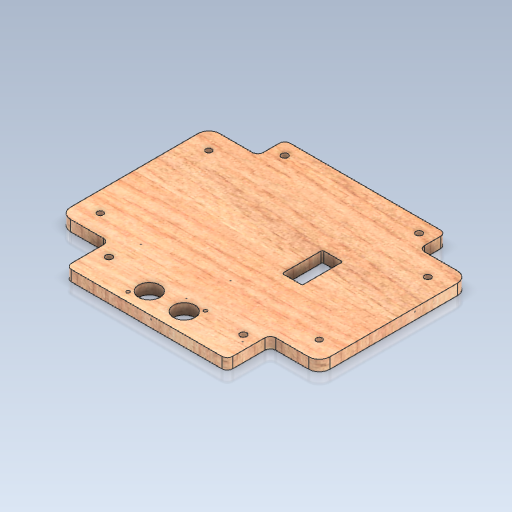
# Autodesk Inventor part: lcd mount back
Saved by Autodesk Inventor 2020.2 (Build 242310000, 310)
## iProperties
Created: 2019-10-18
Part Number: lcd mount back
Material: Wood (Birch)
Document SubType Name: Modeling
Designer: Stefan de Kraker
Density: 0.55 g/cm^3
Appearance: Birch - Natural Polished
Author: Stefan de Kraker
Autodesk Inventor part; units mm, degrees
ref_plane "YZ Plane" through (0, 0, 0) normal (1, 0, 0) x (0, 1, 0)
ref_plane "XZ Plane" through (0, 0, 0) normal (0, 1, 0) x (-1, 0, 0)
ref_plane "XY Plane" through (0, 0, 0) normal (0, 0, 1) x (1, 0, 0)
sketch "Sketch1" plane through (0, 0, 0) normal (0, 1, 0) x (-1, 0, 0)
  arc A0 (0, 0) -> (-7.88, -7.88) centre (0, -7.88) ccw
  line L0 (177.2, 0) -> (0, 0)
  arc A1 (185.08, -7.88) -> (177.2, 0) centre (177.2, -7.88) ccw
  arc A2 (177.2, -110.76) -> (185.08, -102.88) centre (177.2, -102.88) ccw
  line L1 (185.08, -102.88) -> (185.08, -7.88)
  line L2 (0, -110.76) -> (177.2, -110.76)
  line L3 (-7.88, -7.88) -> (-7.88, -102.88)
  arc A3 (-7.88, -102.88) -> (0, -110.76) centre (0, -102.88) ccw
  line L4 (63.5998, -43.83) -> (48.5998, -43.83)
  line L5 (48.5998, -43.83) -> (48.5998, -73.83)
  line L6 (48.5998, -73.83) -> (63.5998, -73.83)
  line L7 (63.5998, -73.83) -> (63.5998, -43.83)
  line L8 (138.6, 10) -> (38.6, 10)
  line L9 (38.6, 10) -> (38.6, -120.76)
  line L10 (38.6, -120.76) -> (138.6, -120.76)
  line L11 (138.6, -120.76) -> (138.6, 10)
  line L12 (148.6, 20) -> (28.6, 20)
  line L13 (28.6, 20) -> (28.6, -130.76)
  line L14 (28.6, -130.76) -> (148.6, -130.76)
  line L15 (148.6, -130.76) -> (148.6, 20)
  line L16 (114.72, -33.83) -> (114.72, -83.83) projected
  arc A4 (111.72, -86.83) -> (114.72, -83.83) centre (111.72, -83.83) ccw projected
  line L17 (111.72, -86.83) -> (52.72, -86.83) projected
  arc A5 (49.72, -83.83) -> (52.72, -86.83) centre (52.72, -83.83) ccw projected
  line L18 (49.72, -83.83) -> (49.72, -33.83) projected
  arc A6 (52.72, -30.83) -> (49.72, -33.83) centre (52.72, -33.83) ccw projected
  line L19 (52.72, -30.83) -> (111.72, -30.83) projected
  arc A7 (114.72, -33.83) -> (111.72, -30.83) centre (111.72, -33.83) ccw projected
  circle A8 centre (53.22, -83.33) radius 1.375 projected
  circle A9 centre (111.22, -83.33) radius 1.375 projected
  circle A10 centre (53.22, -34.33) radius 1.375 projected
  circle A11 centre (111.22, -34.33) radius 1.375 projected
  point P0 (63.5998, -58.83)
  point P1 (185.08, -55.38)
  point P2 (88.6, 10)
  point P3 (88.6, 0)
  point P4 (33.6, -43.83)
  point P5 (33.6, -73.83)
  point P6 (28.6, -110.76)
  point P7 (148.6, -110.76)
  point P8 (148.6, 0)
  point P9 (28.6, 0)
  dimension "d2" = 30
  dimension "d3" = 15
  dimension "d5" = 100
  dimension "d6" = 10
  dimension "d7" = 10
  dimension "d8" = 10
  dimension "d17" = 13
  dimension "d37" = 56.4798
  constraints: 32 end point, 8 point on circle, 6 parallel, 4 centre point, 4 coincident, 4 midpoint, 3 perpendicular, 2 horizontal, 1 vertical alignment, 3 other
  measures "d2" distance of L6.end L4.start
  measures "d3" distance of L5.end L6.end
  measures "d5" distance of L9.end L10.end
  measures "d6" distance between parallel lines of L2 L10
  measures "d7" distance between parallel lines of L0 L8
  measures "d8" distance between parallel lines of L11 L15
  measures "d17" distance between parallel lines of L6 L17
  measures "d37" distance between parallel lines of L3 L5
extrude "Extrusion1" add sketch "Sketch1" along normal blind 8 contours L0 L13 L2 A3 L3 A0 | L13 L12 L15 L0 L11 L8 L9 | L0 L9 L2 L13 | L9 L8 L11 L0 | L0 L11 L2 L9 | L2 L9 L10 L11 L15 L14 L13 | L0 L15 L2 L11 | L2 L11 L10 L9 | L0 A1 L1 A2 L2 L15 | L4 L18 A6 L19 A7 L16 A4 L17 A5 L6 L7 | A8 | A9 | A10 | A11
hole "Hole1" at (-138.6, 0, 10) at (-38.6, 0, 10) at (-38.6, 0, -120.76) at (-138.6, 0, -120.76) direction (0, 1, 0) diameter 5 end through all
fillet "Fillet1" radius 4 8 edges at (-28.6, 4, -110.76) (-28.6, 4, -130.76) (-148.6, 4, -110.76) (-148.6, 4, -130.76) (-148.6, 4, 0) (-148.6, 4, 20) (-28.6, 4, 20) (-28.6, 4, 0)
fillet "Fillet2" radius 1 4 edges at (-63.5998, 4, -73.83) (-48.5998, 4, -73.83) (-48.5998, 4, -43.83) (-63.5998, 4, -43.83)
move faces "Move1" translate (0, 0, 12) faces at (-107.2667, 2.6667, 20)
sketch "Sketch2" plane through (0, 0, 0) normal (0, -1, 0) x (1, 0, 0)
  circle A0 centre (-109.1, 25.25) radius 1.25
  circle A1 centre (-101.6, 17) radius 8
  circle A2 centre (-75.6, 17) radius 8
  circle A3 centre (-68.1, 8.75) radius 1.25
  line L0 (-101.6, 17) -> (-75.6, 17)
  line L1 (-144.6, 32) -> (-32.6, 32) projected
  line L2 (-32.6, -130.76) -> (-144.6, -130.76) projected
  point P0 (0, 0)
  point P1 (0, 0)
  point P2 (-88.6, 17)
  point P3 (-88.6, -130.76)
  point P4 (-88.6, 32)
  dimension "d24" = 26
  dimension "d28" = 16
  dimension "d29" = 16
  dimension "d34" = 15
  dimension "d38" = 7.5
  dimension "d40" = 41
  dimension "d41" = 16.5
  dimension "d42" = 8.25
  constraints: 4 centre point, 3 midpoint, 2 end point, 2 vertical alignment, 1 horizontal, 1 horizontal alignment
  measures "d24" distance of L0.end L0.start
  measures "d28" diameter of A2
  measures "d29" diameter of A1
  measures "d34" distance between parallel lines of L1 L0
  measures "d38" horizontal distance of A3.centre L0.end
  measures "d40" horizontal distance of A0.centre A3.centre
  measures "d41" vertical distance of A3.centre A0.centre
  measures "d42" vertical distance of L0.start A0.centre
extrude "Extrusion2" cut sketch "Sketch2" against normal through all
sketch "Sketch3" plane through (0, 0, 0) normal (0, -1, 0) x (1, 0, 0)
  line L0 (-16.12, -20) -> (-161.08, -20) projected
  arc A0 (-161.08, -20) -> (-165.08, -24) centre (-161.08, -24) ccw projected
  line L1 (-165.08, -24) -> (-165.08, -86.76) projected
  arc A1 (-165.08, -86.76) -> (-161.08, -90.76) centre (-161.08, -86.76) ccw projected
  line L2 (-161.08, -90.76) -> (-16.12, -90.76) projected
  arc A2 (-16.12, -90.76) -> (-12.12, -86.76) centre (-16.12, -86.76) ccw projected
  line L3 (-12.12, -86.76) -> (-12.12, -24) projected
  arc A3 (-12.12, -24) -> (-16.12, -20) centre (-16.12, -24) ccw projected
  line L4 (-10.8728, -95.76) -> (-8.9964, -99.01) projected
  line L5 (-8.9964, -99.01) -> (-5.2436, -99.01) projected
  line L6 (-5.2436, -99.01) -> (-3.3672, -95.76) projected
  line L7 (-3.3672, -95.76) -> (-5.2436, -92.51) projected
  line L8 (-5.2436, -92.51) -> (-8.9964, -92.51) projected
  line L9 (-8.9964, -92.51) -> (-10.8728, -95.76) projected
  line L10 (-168.2036, -11.75) -> (-171.9564, -11.75) projected
  line L11 (-171.9564, -11.75) -> (-173.8328, -15) projected
  line L12 (-173.8328, -15) -> (-171.9564, -18.25) projected
  line L13 (-171.9564, -18.25) -> (-168.2036, -18.25) projected
  line L14 (-168.2036, -18.25) -> (-166.3272, -15) projected
  line L15 (-166.3272, -15) -> (-168.2036, -11.75) projected
  line L16 (-5.2436, -18.25) -> (-3.3672, -15) projected
  line L17 (-3.3672, -15) -> (-5.2436, -11.75) projected
  line L18 (-5.2436, -11.75) -> (-8.9964, -11.75) projected
  line L19 (-8.9964, -11.75) -> (-10.8728, -15) projected
  line L20 (-10.8728, -15) -> (-8.9964, -18.25) projected
  line L21 (-8.9964, -18.25) -> (-5.2436, -18.25) projected
  line L22 (-173.8328, -95.76) -> (-171.9564, -99.01) projected
  line L23 (-171.9564, -99.01) -> (-168.2036, -99.01) projected
  line L24 (-168.2036, -99.01) -> (-166.3272, -95.76) projected
  line L25 (-166.3272, -95.76) -> (-168.2036, -92.51) projected
  line L26 (-168.2036, -92.51) -> (-171.9564, -92.51) projected
  line L27 (-171.9564, -92.51) -> (-173.8328, -95.76) projected
  arc A4 (7.88, -7.88) -> (0, 0) centre (0, -7.88) ccw projected
  line L28 (7.88, -102.88) -> (7.88, -7.88) projected
  arc A5 (0, -110.76) -> (7.88, -102.88) centre (0, -102.88) ccw projected
  line L29 (-177.2, -110.76) -> (0, -110.76) projected
  arc A6 (-185.08, -102.88) -> (-177.2, -110.76) centre (-177.2, -102.88) ccw projected
  line L30 (-185.08, -7.88) -> (-185.08, -102.88) projected
  arc A7 (-177.2, 0) -> (-185.08, -7.88) centre (-177.2, -7.88) ccw projected
  line L31 (0, 0) -> (-177.2, 0) projected
  circle A8 centre (-7.12, -95.76) radius 2.4
  circle A9 centre (-170.08, -95.76) radius 2.25
  circle A10 centre (-170.08, -15) radius 2.25
  circle A11 centre (-7.12, -15) radius 2.25
  dimension "d43" = 4.8
  dimension "d44" = 4.5
  dimension "d45" = 4.5
  dimension "d46" = 4.5
  constraints: 4 centre point
  measures "d43" diameter of A8
  measures "d44" diameter of A9
  measures "d45" diameter of A10
  measures "d46" diameter of A11
extrude "Extrusion3" cut sketch "Sketch3" against normal through all contours A8 | A9 | A10 | A11
equation "\"d42\" = 0.5 * d41"
body "Solid1"
